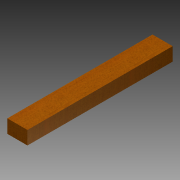
# Autodesk Inventor part: Tower_Out
Saved by Autodesk Inventor 2014 SP1 (Build 180222100, 222)
## iProperties
Created: 2014-02-22
Part Number: Tower_Out
Material: Wood
Document SubType Name: Modeling
Designer: tuleu
Density: 0.570257 g/cm^3
Appearance: Yellow Pine - Solid Natural Low Gloss
Author: tuleu
Autodesk Inventor part; units mm, degrees
ref_plane "YZ Plane" through (0, 0, 0) normal (1, 0, 0) x (0, 1, 0)
ref_plane "XZ Plane" through (0, 0, 0) normal (0, 1, 0) x (-1, 0, 0)
ref_plane "XY Plane" through (0, 0, 0) normal (0, 0, 1) x (1, 0, 0)
sketch "Sketch1" plane through (0, 0, 0) normal (0, 0, 1) x (1, 0, 0)
  line L0 (-100, 463) -> (-60, 463) construction
  line L1 (-60, 463) -> (631.4317, 463) construction
  line L2 (613, 30) -> (553, 30)
  line L3 (553, 30) -> (553, 463)
  line L4 (553, 463) -> (613, 463)
  line L5 (613, 463) -> (613, 30)
  point P0 (0, 0)
  dimension "d0" = 60
  constraints: 10 end point, 2 parallel, 1 collinear, 1 horizontal, 1 perpendicular, 1 point on line, 1 other
  measures "d0" distance between parallel lines of L5 L3
extrude "Extrusion1" add sketch "Sketch1" against normal blind 40
body "Solid1"
